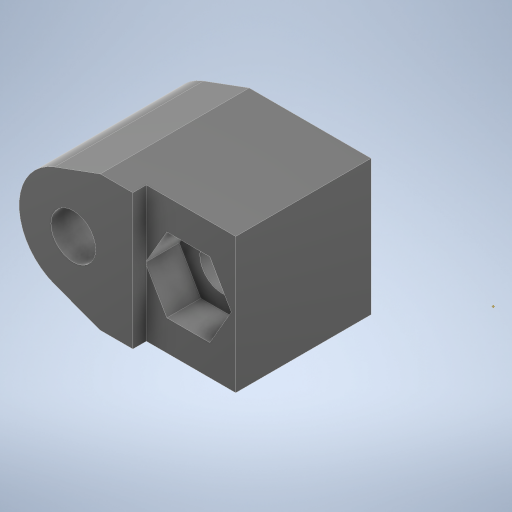
# Autodesk Inventor part: power_signal_socket_fixed3
Saved by Autodesk Inventor 2023 (Build 270158000, 158)
## iProperties
Created: 2023-09-07
Part Number: power_signal_socket_fixed3
Material: Acetal Resin, Black
Document SubType Name: Modeling
Designer: 310611102
Density: 1.425 g/cm^3
Appearance: Smooth - Black
Mass: 1.68612 g
Surface Area: 9.54326 cm^2
Volume: 1.18324 cm^3
Author: 310611102
Autodesk Inventor part; units mm, degrees
ref_plane "YZ Plane" through (0, 0, 0) normal (1, 0, 0) x (0, 1, 0)
ref_plane "XZ Plane" through (0, 0, 0) normal (0, 1, 0) x (-1, 0, 0)
ref_plane "XY Plane" through (0, 0, 0) normal (0, 0, 1) x (1, 0, 0)
sketch "Sketch2" plane through (0, 0, 0) normal (0, 0, 1) x (1, 0, 0)
  line L0 (-18, 5) -> (18, 5)
  line L1 (18, 5) -> (18, -5)
  line L2 (18, -5) -> (-18, -5)
  line L3 (-18, -5) -> (-18, 5)
  line L4 (-18, 5) -> (18, -5) construction
  line L5 (18, 5) -> (-18, -5) construction
  point P0 (0, 0)
  dimension "d0" = 10
  dimension "d1" = 36
  constraints: 12 end point, 2 midpoint, 2 parallel, 1 horizontal, 1 perpendicular
  measures "d0" distance of L0.end L1.end
  measures "d1" distance of L0.start L0.end
extrude "Extrusion1" add sketch "Sketch2" along normal blind 11
sketch "Sketch3" plane through (0, 0, 11) normal (0, 0, 1) x (1, 0, 0)
  line L0 (-15.6, 12.15) -> (15.6, 12.15)
  line L1 (15.6, 12.15) -> (15.6, -12.15)
  line L2 (15.6, -12.15) -> (-15.6, -12.15)
  line L3 (-15.6, -12.15) -> (-15.6, 12.15)
  line L4 (-15.6, 12.15) -> (15.6, -12.15) construction
  line L5 (15.6, 12.15) -> (-15.6, -12.15) construction
  point P0 (0, 0)
  dimension "d4" = 31.2
  dimension "d5" = 24.3
  constraints: 12 end point, 2 midpoint, 2 parallel, 1 horizontal, 1 perpendicular
  measures "d4" distance of L0.start L0.end
  measures "d5" distance of L0.end L1.end
extrude "Extrusion2" cut sketch "Sketch3" against normal blind 1
sketch "Sketch4" plane through (0, 0, 10) normal (0, 0, 1) x (1, 0, 0)
  circle A0 centre (12.5, 0) radius 1.65
  line L0 (0, 0) -> (0, 4.6535) construction
  circle A1 centre (-12.5, 0) radius 1.65
  point P0 (-61.5247, -30.2854)
  point P1 (15.4586, -30.2854)
  dimension "d39" = 3.3
  dimension "d40" = 25
  constraints: 2 centre point, 2 end point, 1 horizontal alignment, 1 symmetric about line, 1 vertical, 1 other
  measures "d39" diameter of A0
  measures "d40" distance of A0.centre A1.centre
extrude "Extrusion3" cut sketch "Sketch4" against normal through all
sketch "Sketch7" plane through (0, 0, 11) normal (0, 0, 1) x (1, 0, 0)
  arc A0 (21.3831, -3.7533) -> (21.3831, 3.7533) centre (20, 0) ccw
  line L0 (21.3831, 3.7533) -> (18, 5)
  line L1 (18, 5) -> (18, -5)
  line L2 (18, -5) -> (21.3831, -3.7533)
  line L3 (0, 20.7674) -> (0, -20.7674) construction
  arc A1 (-21.3831, 3.7533) -> (-21.3831, -3.7533) centre (-20, 0) ccw
  line L4 (-21.3831, 3.7533) -> (-18, 5)
  line L5 (-18, 5) -> (-18, -5)
  line L6 (-18, -5) -> (-21.3831, -3.7533)
  line L7 (18, -5) -> (18, 5) construction
  circle A2 centre (20, 0) radius 1.65
  circle A3 centre (-20, 0) radius 1.65
  line L8 (0, 0) -> (1.9739, 0) construction
  dimension "d28" = 3.3
  dimension "d29" = 4
  dimension "d30" = 40
  dimension "d31" = 10
  constraints: 16 end point, 6 symmetric about line, 4 centre point, 4 point on circle, 2 coincident, 2 tangent, 1 horizontal, 1 horizontal alignment, 1 midpoint, 1 point on line, 1 vertical, 3 other
  measures "d28" diameter of A2
  measures "d29" radius of A0
  measures "d30" distance of A1.centre A0.centre
  measures "d31" distance of L0.end L1.end
extrude "Extrusion6" add sketch "Sketch7" against normal up to surface (11 mm away)
sketch "Sketch9" plane through (0, 0, 10) normal (0, 0, 1) x (1, 0, 0)
  circle A0 centre (-12.5, 0) radius 1.65 projected
  line L0 (-9.3246, 0) -> (-10.9123, -2.75)
  line L1 (-10.9123, -2.75) -> (-14.0877, -2.75)
  line L2 (-14.0877, -2.75) -> (-15.6754, 0)
  line L3 (-15.6754, 0) -> (-14.0877, 2.75)
  line L4 (-14.0877, 2.75) -> (-10.9123, 2.75)
  line L5 (-10.9123, 2.75) -> (-9.3246, 0)
  line L6 (0, 0) -> (0, 3.6506) construction
  circle A1 centre (12.5, 0) radius 1.65
  line L7 (9.3246, 0) -> (10.9123, -2.75)
  line L8 (10.9123, -2.75) -> (14.0877, -2.75)
  line L9 (14.0877, -2.75) -> (15.6754, 0)
  line L10 (15.6754, 0) -> (14.0877, 2.75)
  line L11 (14.0877, 2.75) -> (10.9123, 2.75)
  line L12 (10.9123, 2.75) -> (9.3246, 0)
  dimension "d41" = 5.5
  constraints: 26 end point, 8 symmetric about line, 2 coincident, 1 centre point, 1 horizontal, 1 vertical, 14 other
  measures "d41" distance between parallel lines of L1 L4
extrude "Extrusion8" cut sketch "Sketch9" against normal blind 2.5
sketch "Sketch8" plane through (0, 0, 0) normal (1, 0, 0) x (0, 1, 0)
  line L0 (45.1511, -28.2394) -> (-45.1511, -28.2394)
  line L1 (-45.1511, -28.2394) -> (-45.1511, 28.2394)
  line L2 (-45.1511, 28.2394) -> (45.1511, 28.2394)
  line L3 (45.1511, 28.2394) -> (45.1511, -28.2394)
  line L4 (45.1511, -28.2394) -> (-45.1511, 28.2394) construction
  line L5 (-45.1511, -28.2394) -> (45.1511, 28.2394) construction
  point P0 (0, 0)
  constraints: 12 end point, 2 midpoint, 2 parallel, 1 horizontal, 1 perpendicular
extrude "Extrusion7" cut sketch "Sketch8" along normal blind 24 and the other way blind 9
body "Solid1"
